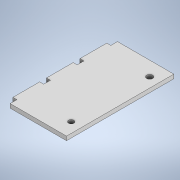
# Autodesk Inventor part: Part2
Saved by Autodesk Inventor 2022 (Build 260153000, 153)
## iProperties
Created: 2021-10-21
Part Number: Part2
Material: Generic
Document SubType Name: Modeling
Designer: Administrador
Density: 1 g/cm^3
Appearance: Default
Author: Administrador
Autodesk Inventor part; units mm, degrees
ref_plane "YZ Plane" through (0, 0, 0) normal (1, 0, 0) x (0, 1, 0)
ref_plane "XZ Plane" through (0, 0, 0) normal (0, 1, 0) x (-1, 0, 0)
ref_plane "XY Plane" through (0, 0, 0) normal (0, 0, 1) x (1, 0, 0)
sketch "Sketch1" plane through (0, 0, 0) normal (0, 1, 0) x (-1, 0, 0)
  line L0 (0, 0) -> (-42, 0)
  line L1 (-42, 0) -> (-42, -80)
  line L2 (-42, -80) -> (0, -80)
  line L3 (0, 0) -> (0, -5)
  line L4 (0, -5) -> (3, -5)
  line L5 (3, -5) -> (3, -25)
  line L6 (3, -25) -> (0, -25)
  line L7 (0, -80) -> (0, -75)
  line L8 (0, -75) -> (3, -75)
  line L9 (3, -75) -> (3, -55)
  line L10 (3, -55) -> (0, -55)
  line L11 (0, -25) -> (0, -30)
  line L12 (0, -30) -> (3, -30)
  line L13 (3, -30) -> (3, -50)
  line L14 (3, -50) -> (0, -50)
  line L15 (0, -50) -> (0, -55)
  line L16 (0, -40) -> (0, -13) construction
  line L17 (0, -13) -> (-32.5, -13) construction
  line L18 (-32.5, -13) -> (-36.5, -13) construction
  line L19 (-36.5, -13) -> (-36.5, -9) construction
  line L20 (-36.5, -9) -> (-32.5, -9) construction
  line L21 (-32.5, -9) -> (-32.5, -13) construction
  circle A0 centre (-34.5, -11) radius 2
  line L22 (-32.5, -13) -> (-32.5, -67) construction
  line L23 (-32.5, -67) -> (-37, -67) construction
  line L24 (-37, -67) -> (-37, -71.5) construction
  line L25 (-37, -71.5) -> (-32.5, -71.5) construction
  line L26 (-32.5, -71.5) -> (-32.5, -67) construction
  circle A1 centre (-34.75, -69.25) radius 2.25
  point P0 (-36.5, -11)
  point P1 (-37, -69.25)
  dimension "d1" = 80
  dimension "d2" = 5
  dimension "d3" = 3
  dimension "d4" = 20
  dimension "d5" = 5
  dimension "d6" = 20
  dimension "d7" = 5
  dimension "d8" = 20
  dimension "d12" = 27
  dimension "d13" = 32.5
  dimension "d14" = 4
  dimension "d15" = 4
  dimension "d16" = 54
  dimension "d17" = 4.5
  dimension "d18" = 4.5
  dimension "d20" = 5
  dimension "d21" = 0
  dimension "d22" = 3
  dimension "d23" = 0
  constraints: 54 end point, 8 parallel, 7 horizontal, 6 perpendicular, 3 vertical, 2 horizontal alignment, 2 midpoint, 4 other
  measures "d1" distance of L1.end L0.end
  measures "d2" distance of L0.start L3.end
  measures "d3" distance of L5.end L6.end
  measures "d4" distance of L4.end L5.end
  measures "d5" distance of L2.end L7.end
  measures "d6" distance of L9.end L8.end
  measures "d7" distance of L6.end L11.end
  measures "d8" distance of L12.end L13.end
  measures "d12" distance of L16.start L16.end
  measures "d13" distance of L16.end L17.end
  measures "d14" distance of L19.end L20.end
  measures "d15" distance of L18.end L19.end
  measures "d16" distance of L17.end L22.end
  measures "d17" distance of L25.end L24.end
  measures "d18" distance of L24.end L23.end
  measures "d20" distance from line of L1 point (-37, -69.25)
  measures "d21" distance between parallel lines of L16 L15
  measures "d22" distance between parallel lines of L15 L9
  measures "d23" distance between parallel lines of L15 L7
extrude "Extrusion1" add sketch "Sketch1" along normal blind 3
body "Solid1"
